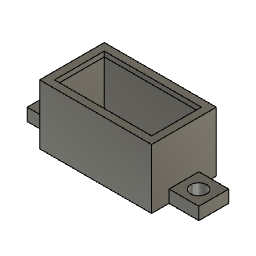
Relais-Holder (Autodesk Fusion 360 design; units mm, degrees)
Autodesk Fusion 360 part; units mm, degrees
sketch "Sketch2" plane through (0, 0, 0) normal (0, 0, 1) x (1, 0, 0)
  line L0 (0, 0) -> (20.5, 0)
  line L1 (20.5, 0) -> (20.5, 11)
  line L2 (20.5, 11) -> (0, 11)
  line L3 (0, 11) -> (0, 0)
  line L4 (-1, -1) -> (21.5, -1)
  line L5 (21.5, -1) -> (21.5, 12)
  line L6 (21.5, 12) -> (-1, 12)
  line L7 (-1, 12) -> (-1, -1)
  line L8 (-1, 5.5) -> (21.5, 5.5) construction
  line L9 (-1, 2.5) -> (-7, 2.5)
  line L10 (-7, 2.5) -> (-7, 8.5)
  line L11 (-7, 8.5) -> (-1, 8.5)
  line L12 (-1, 8.5) -> (-1, 2.5)
  line L13 (10.25, 12) -> (10.25, -1) construction
  circle A0 centre (-4.0214, 5.4305) radius 1.6
  circle A1 centre (24.5214, 5.4305) radius 1.6
  line L14 (27.5, 8.5) -> (21.5, 8.5)
  line L15 (27.5, 2.5) -> (27.5, 8.5)
  line L16 (21.5, 2.5) -> (27.5, 2.5)
  dimension "d1" = 20.5
  dimension "d2" = 11
  dimension "d3" = 1
  dimension "d9" = 3.2
  dimension "d10" = 6
  dimension "d11" = 6
  constraint horizontal L0
  constraint vertical L1
  constraint horizontal L2
  constraint vertical L3
  constraint coincident L0.start L3.end
  constraint midpoint L7 L8.start
  constraint midpoint L5 L8.end
  constraint horizontal L9
  constraint vertical L10
  constraint horizontal L11
  constraint vertical L12
  constraint coincident L7 L9.start
  constraint symmetric L8 L9 L11
  constraint midpoint L6 L13.start
  constraint midpoint L4 L13.end
  constraint symmetric L9.start L13 L16.start
  constraint symmetric L9.end L13 L15.start
  constraint symmetric L10.end L13 L14.start
  constraint symmetric L11.end L13 L14.end
  constraint symmetric L13 A0 A1
  measures "d1" distance of L0.start L0.end
  measures "d2" distance of L0.start L2.end
  measures "d9" diameter of A0
  measures "d10" distance of L9.end L10.end
  measures "d11" distance of L7 L10
extrude "Extrude3" add sketch "Sketch2" along normal blind 2.5 contours L7 L9 L10 L11 L12 | L5 L14 L15 L16 makes body 1 at (-4.047, 8.0087, 0) makes body 2 at (24.4673, 8.0087, 0)
extrude "Extrude1" add sketch "Sketch2" along normal blind 11 separate body contours L4 L5 L6 L7 L12 makes body 3
sketch "Sketch3" plane through (0, 0, 11) normal (0, 0, 1) x (-1, 0, 0)
  line L0 (0, 0) -> (0, -11)
  line L1 (0, -11) -> (-20.5, -11)
  line L2 (-20.5, -11) -> (-20.5, 0)
  line L3 (-20.5, 0) -> (0, 0)
  line L4 (1, -12) -> (1, 1)
  line L5 (1, 1) -> (-21.5, 1)
  line L6 (-21.5, 1) -> (-21.5, -12)
  line L7 (-21.5, -12) -> (1, -12)
  line L8 (-20, -0.5) -> (-0.5, -0.5)
  line L9 (-0.5, -0.5) -> (-0.5, -10.5)
  line L10 (-0.5, -10.5) -> (-20, -10.5)
  line L11 (-20, -10.5) -> (-20, -0.5)
  dimension "d6" = 0.5
extrude "Extrude2" add sketch "Sketch3" along normal blind 1 contours L0 L1 L2 L3 | L4 L5 L6 L7 bodies 3
